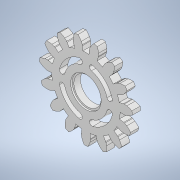
# Autodesk Inventor part: ｍ2歯数15ギア3td3.99
Saved by Autodesk Inventor 2020.2 (Build 242310000, 310)
## iProperties
Created: 2020-03-08
Part Number: ｍ2歯数15ギア3td3.99
Material: アルミニウム 2014-T4
Document SubType Name: Modeling
Designer: aoyam
Density: 2.8 g/cm^3
Appearance: サテン
Author: aoyam
Autodesk Inventor part; units mm, degrees
ref_plane "YZ Plane" through (0, 0, 0) normal (1, 0, 0) x (0, 1, 0)
ref_plane "XZ Plane" through (0, 0, 0) normal (0, 1, 0) x (-1, 0, 0)
ref_plane "XY Plane" through (0, 0, 0) normal (0, 0, 1) x (1, 0, 0)
sketch "スケッチ1" plane through (0, 0, 0) normal (0, 0, 1) x (1, 0, 0)
  arc A0 (3.0837, 16.0363) -> (3.0209, 15.76) centre (4.5944, 15.5478) ccw
  arc A1 (3.4621, 16.9034) -> (3.0837, 16.0363) centre (7.2791, 14.7216) ccw
  arc A2 (4.6507, 18.4808) -> (3.4621, 16.9034) centre (10.1692, 13.0859) ccw
  arc A3 (0.486, 15.76) -> (0.4232, 16.0363) centre (-1.0874, 15.5478) ccw
  arc A4 (0.4232, 16.0363) -> (0.0449, 16.9034) centre (-3.7722, 14.7216) ccw
  arc A5 (0.0449, 16.9034) -> (-1.1438, 18.4808) centre (-6.6623, 13.0859) ccw
  arc A6 (2.8775, 14.1671) -> (0.6295, 14.1671) centre (1.7535, 1.6862) ccw
  arc A7 (-1.1438, 18.4808) -> (-2.4308, 18.2073) centre (1.7535, 1.6862) ccw
  line L0 (2.8775, 14.1671) -> (3.0209, 15.76)
  line L1 (0.6295, 14.1671) -> (0.486, 15.76)
  line L2 (-4.3498, 12.6309) -> (-5.1288, 14.0278)
  arc A8 (-5.1288, 14.0278) -> (-5.2985, 14.2546) centre (-6.4799, 13.1939) ccw
  arc A9 (-5.2985, 14.2546) -> (-5.9968, 14.8928) centre (-8.5965, 11.3472) ccw
  arc A10 (-5.9968, 14.8928) -> (-7.7243, 15.8504) centre (-10.5714, 8.6774) ccw
  arc A11 (-7.7243, 15.8504) -> (-8.7887, 15.0771) centre (1.7535, 1.6862) ccw
  arc A12 (-2.868, 15.3367) -> (-2.813, 15.0588) centre (-1.2893, 15.5049) ccw
  arc A13 (-2.2961, 13.5452) -> (-4.3498, 12.6309) centre (1.7535, 1.6862) ccw
  line L3 (-2.2961, 13.5452) -> (-2.813, 15.0588)
  arc A14 (-2.875, 16.2827) -> (-2.868, 15.3367) centre (1.4994, 15.8421) ccw
  arc A15 (-2.4308, 18.2073) -> (-2.875, 16.2827) centre (4.805, 15.5234) ccw
  line L4 (-8.2737, 9.2022) -> (-9.5535, 10.1615)
  arc A16 (-9.5535, 10.1615) -> (-9.8008, 10.2997) centre (-10.4487, 8.8502) ccw
  arc A17 (-9.8008, 10.2997) -> (-10.6984, 10.5987) centre (-11.6311, 6.3022) ccw
  arc A18 (-10.6984, 10.5987) -> (-12.666, 10.7709) centre (-12.3494, 3.06) ccw
  arc A19 (-12.666, 10.7709) -> (-13.3239, 9.6314) centre (1.7535, 1.6862) ccw
  arc A20 (-8.0207, 12.2768) -> (-7.8573, 12.0453) centre (-6.6468, 13.0726) ccw
  arc A21 (-6.7695, 10.8728) -> (-8.2737, 9.2022) centre (1.7535, 1.6862) ccw
  line L5 (-6.7695, 10.8728) -> (-7.8573, 12.0453)
  arc A22 (-8.4118, 13.1382) -> (-8.0207, 12.2768) centre (-4.2364, 14.515) ccw
  arc A23 (-8.7887, 15.0771) -> (-8.4118, 13.1382) centre (-1.0869, 15.5682) ccw
  line L6 (-10.4639, 4.474) -> (-12.0232, 4.8298)
  arc A24 (-12.0232, 4.8298) -> (-12.3054, 4.8555) centre (-12.3076, 3.2678) ccw
  arc A25 (-12.3054, 4.8555) -> (-13.2469, 4.7636) centre (-12.3515, 0.4591) ccw
  arc A26 (-13.2469, 4.7636) -> (-15.1145, 4.1206) centre (-11.6889, -2.795) ccw
  arc A27 (-15.1145, 4.1206) -> (-15.252, 2.812) centre (1.7535, 1.6862) ccw
  arc A28 (-11.4832, 7.3857) -> (-11.2399, 7.2407) centre (-10.5518, 8.6715) ccw
  arc A29 (-9.7692, 6.612) -> (-10.4639, 4.474) centre (1.7535, 1.6862) ccw
  line L7 (-9.7692, 6.612) -> (-11.2399, 7.2407)
  arc A30 (-12.1909, 8.0135) -> (-11.4832, 7.3857) centre (-8.9365, 10.9696) ccw
  arc A31 (-13.3239, 9.6314) -> (-12.1909, 8.0135) centre (-6.4877, 13.2128) ccw
  line L8 (-10.5416, -0.7363) -> (-12.1108, -1.0455)
  arc A32 (-12.1108, -1.0455) -> (-12.379, -1.1368) centre (-11.7353, -2.5881) ccw
  arc A33 (-12.379, -1.1368) -> (-13.2018, -1.6037) centre (-10.633, -5.1718) ccw
  arc A34 (-13.2018, -1.6037) -> (-14.6463, -2.9507) centre (-8.7041, -7.8751) ccw
  arc A35 (-14.6463, -2.9507) -> (-14.2397, -4.2021) centre (1.7535, 1.6862) ccw
  arc A36 (-12.6571, 1.5091) -> (-12.3758, 1.4756) centre (-12.3292, 3.0626) ccw
  arc A37 (-10.7765, 1.4994) -> (-10.5416, -0.7363) centre (1.7535, 1.6862) ccw
  line L9 (-10.7765, 1.4994) -> (-12.3758, 1.4756)
  arc A38 (-13.5589, 1.7948) -> (-12.6571, 1.5091) centre (-11.7881, 5.819) ccw
  arc A39 (-15.252, 2.812) -> (-13.5589, 1.7948) centre (-10.4635, 8.8642) ccw
  line L10 (-8.4933, -5.5277) -> (-9.8011, -6.4484)
  arc A40 (-9.8011, -6.4484) -> (-10.009, -6.6409) centre (-8.8306, -7.705) ccw
  arc A41 (-10.009, -6.6409) -> (-10.5707, -7.4021) centre (-6.7727, -9.6169) ccw
  arc A42 (-10.5707, -7.4021) -> (-11.3425, -9.2202) centre (-3.9111, -11.302) ccw
  arc A43 (-11.3425, -9.2202) -> (-10.4621, -10.198) centre (1.7535, 1.6862) ccw
  arc A44 (-11.3392, -4.3369) -> (-11.0686, -4.2531) centre (-11.6715, -2.7843) ccw
  arc A45 (-9.6173, -3.5809) -> (-8.4933, -5.5277) centre (1.7535, 1.6862) ccw
  line L11 (-9.6173, -3.5809) -> (-11.0686, -4.2531)
  arc A46 (-12.2793, -4.4427) -> (-11.3392, -4.3369) centre (-12.2984, -0.0462) ccw
  arc A47 (-14.2397, -4.2021) -> (-12.2793, -4.4427) centre (-12.3269, 3.2746) ccw
  line L12 (-4.6733, -9.0717) -> (-5.4935, -10.4448)
  arc A48 (-5.4935, -10.4448) -> (-5.6051, -10.7052) centre (-4.0958, -11.198) ccw
  arc A49 (-5.6051, -10.7052) -> (-5.8087, -11.6291) centre (-1.4382, -12.1076) ccw
  arc A50 (-5.8087, -11.6291) -> (-5.7743, -13.6039) centre (1.8614, -12.4831) ccw
  arc A51 (-5.7743, -13.6039) -> (-4.5723, -14.1391) centre (1.7535, 1.6862) ccw
  arc A52 (-7.7575, -9.1414) -> (-7.5443, -8.9548) centre (-8.6925, -7.8583) ccw
  arc A53 (-6.4919, -7.7504) -> (-4.6733, -9.0717) centre (1.7535, 1.6862) ccw
  line L13 (-6.4919, -7.7504) -> (-7.5443, -8.9548)
  arc A54 (-8.5732, -9.6205) -> (-7.7575, -9.1414) centre (-10.3789, -5.6118) ccw
  arc A55 (-10.4621, -10.198) -> (-8.5732, -9.6205) centre (-11.7556, -2.5898) ccw
  line L14 (0.258, -10.7557) -> (0.0671, -12.3436)
  arc A56 (0.0671, -12.3436) -> (0.0711, -12.6269) centre (1.6503, -12.4632) ccw
  arc A57 (0.0711, -12.6269) -> (0.2609, -13.5537) centre (4.4482, -12.2133) ccw
  arc A58 (0.2609, -13.5537) -> (1.0956, -15.3438) centre (7.6152, -11.2142) ccw
  arc A59 (1.0956, -15.3438) -> (2.4114, -15.3438) centre (1.7535, 1.6862) ccw
  arc A60 (-2.5312, -12.0738) -> (-2.4124, -11.8166) centre (-3.9074, -11.2819) ccw
  arc A61 (-1.9409, -10.2883) -> (0.258, -10.7557) centre (1.7535, 1.6862) ccw
  line L15 (-1.9409, -10.2883) -> (-2.4124, -11.8166)
  arc A62 (-3.0816, -12.8432) -> (-2.5312, -12.0738) centre (-6.3616, -9.9156) ccw
  arc A63 (-4.5723, -14.1391) -> (-3.0816, -12.8432) centre (-8.8485, -7.7147) ccw
  line L16 (5.4478, -10.2883) -> (5.9194, -11.8166)
  arc A64 (5.9194, -11.8166) -> (6.0382, -12.0738) centre (7.4143, -11.2819) ccw
  arc A65 (6.0382, -12.0738) -> (6.5886, -12.8432) centre (9.8686, -9.9156) ccw
  arc A66 (6.5886, -12.8432) -> (8.0792, -14.1391) centre (12.3555, -7.7147) ccw
  arc A67 (8.0792, -14.1391) -> (9.2812, -13.6039) centre (1.7535, 1.6862) ccw
  arc A68 (3.4359, -12.6269) -> (3.4398, -12.3436) centre (1.8566, -12.4632) ccw
  arc A69 (3.249, -10.7557) -> (5.4478, -10.2883) centre (1.7535, 1.6862) ccw
  line L17 (3.249, -10.7557) -> (3.4398, -12.3436)
  arc A70 (3.2461, -13.5537) -> (3.4359, -12.6269) centre (-0.9412, -12.2133) ccw
  arc A71 (2.4114, -15.3438) -> (3.2461, -13.5537) centre (-4.1082, -11.2142) ccw
  line L18 (9.9989, -7.7504) -> (11.0513, -8.9548)
  arc A72 (11.0513, -8.9548) -> (11.2644, -9.1414) centre (12.1995, -7.8583) ccw
  arc A73 (11.2644, -9.1414) -> (12.0802, -9.6205) centre (13.8859, -5.6118) ccw
  arc A74 (12.0802, -9.6205) -> (13.969, -10.198) centre (15.2626, -2.5898) ccw
  arc A75 (13.969, -10.198) -> (14.8494, -9.2202) centre (1.7535, 1.6862) ccw
  arc A76 (9.1121, -10.7052) -> (9.0005, -10.4448) centre (7.6028, -11.198) ccw
  arc A77 (8.1802, -9.0717) -> (9.9989, -7.7504) centre (1.7535, 1.6862) ccw
  line L19 (8.1802, -9.0717) -> (9.0005, -10.4448)
  arc A78 (9.3156, -11.6291) -> (9.1121, -10.7052) centre (4.9452, -12.1076) ccw
  arc A79 (9.2812, -13.6039) -> (9.3156, -11.6291) centre (1.6456, -12.4831) ccw
  line L20 (13.1242, -3.5809) -> (14.5755, -4.2531)
  arc A80 (14.5755, -4.2531) -> (14.8462, -4.3369) centre (15.1785, -2.7843) ccw
  arc A81 (14.8462, -4.3369) -> (15.7862, -4.4427) centre (15.8053, -0.0462) ccw
  arc A82 (15.7862, -4.4427) -> (17.7467, -4.2021) centre (15.8338, 3.2746) ccw
  arc A83 (17.7467, -4.2021) -> (18.1533, -2.9507) centre (1.7535, 1.6862) ccw
  arc A84 (13.5159, -6.6409) -> (13.3081, -6.4484) centre (12.3375, -7.705) ccw
  arc A85 (12.0002, -5.5277) -> (13.1242, -3.5809) centre (1.7535, 1.6862) ccw
  line L21 (12.0002, -5.5277) -> (13.3081, -6.4484)
  arc A86 (14.0777, -7.4021) -> (13.5159, -6.6409) centre (10.2797, -9.6169) ccw
  arc A87 (14.8494, -9.2202) -> (14.0777, -7.4021) centre (7.4181, -11.302) ccw
  line L22 (14.2835, 1.4994) -> (15.8827, 1.4756)
  arc A88 (15.8827, 1.4756) -> (16.164, 1.5091) centre (15.8361, 3.0626) ccw
  arc A89 (16.164, 1.5091) -> (17.0659, 1.7948) centre (15.2951, 5.819) ccw
  arc A90 (17.0659, 1.7948) -> (18.759, 2.812) centre (13.9705, 8.8642) ccw
  arc A91 (18.759, 2.812) -> (18.6214, 4.1206) centre (1.7535, 1.6862) ccw
  arc A92 (15.8859, -1.1368) -> (15.6177, -1.0455) centre (15.2422, -2.5881) ccw
  arc A93 (14.0485, -0.7363) -> (14.2835, 1.4994) centre (1.7535, 1.6862) ccw
  line L23 (14.0485, -0.7363) -> (15.6177, -1.0455)
  arc A94 (16.7087, -1.6037) -> (15.8859, -1.1368) centre (14.1399, -5.1718) ccw
  arc A95 (18.1533, -2.9507) -> (16.7087, -1.6037) centre (12.2111, -7.8751) ccw
  line L24 (13.2762, 6.612) -> (14.7468, 7.2407)
  arc A96 (14.7468, 7.2407) -> (14.9902, 7.3857) centre (14.0588, 8.6715) ccw
  arc A97 (14.9902, 7.3857) -> (15.6979, 8.0135) centre (12.4434, 10.9696) ccw
  arc A98 (15.6979, 8.0135) -> (16.8308, 9.6314) centre (9.9947, 13.2128) ccw
  arc A99 (16.8308, 9.6314) -> (16.173, 10.7709) centre (1.7535, 1.6862) ccw
  arc A100 (15.8123, 4.8555) -> (15.5302, 4.8298) centre (15.8146, 3.2678) ccw
  arc A101 (13.9708, 4.474) -> (13.2762, 6.612) centre (1.7535, 1.6862) ccw
  line L25 (13.9708, 4.474) -> (15.5302, 4.8298)
  arc A102 (16.7539, 4.7636) -> (15.8123, 4.8555) centre (15.8584, 0.4591) ccw
  arc A103 (18.6214, 4.1206) -> (16.7539, 4.7636) centre (15.1959, -2.795) ccw
  line L26 (10.2765, 10.8728) -> (11.3643, 12.0453)
  arc A104 (11.3643, 12.0453) -> (11.5276, 12.2768) centre (10.1537, 13.0726) ccw
  arc A105 (11.5276, 12.2768) -> (11.9188, 13.1382) centre (7.7433, 14.515) ccw
  arc A106 (11.9188, 13.1382) -> (12.2957, 15.0771) centre (4.5939, 15.5682) ccw
  arc A107 (12.2957, 15.0771) -> (11.2312, 15.8504) centre (1.7535, 1.6862) ccw
  arc A108 (13.3078, 10.2997) -> (13.0605, 10.1615) centre (13.9556, 8.8502) ccw
  arc A109 (11.7807, 9.2022) -> (10.2765, 10.8728) centre (1.7535, 1.6862) ccw
  line L27 (11.7807, 9.2022) -> (13.0605, 10.1615)
  arc A110 (14.2053, 10.5987) -> (13.3078, 10.2997) centre (15.1381, 6.3022) ccw
  arc A111 (16.173, 10.7709) -> (14.2053, 10.5987) centre (15.8564, 3.06) ccw
  line L28 (5.8031, 13.5452) -> (6.3199, 15.0588)
  arc A112 (6.3199, 15.0588) -> (6.375, 15.3367) centre (4.7962, 15.5049) ccw
  arc A113 (6.375, 15.3367) -> (6.382, 16.2827) centre (2.0075, 15.8421) ccw
  arc A114 (6.382, 16.2827) -> (5.9377, 18.2073) centre (-1.298, 15.5234) ccw
  arc A115 (5.9377, 18.2073) -> (4.6507, 18.4808) centre (1.7535, 1.6862) ccw
  arc A116 (8.8054, 14.2546) -> (8.6357, 14.0278) centre (9.9868, 13.1939) ccw
  arc A117 (7.8567, 12.6309) -> (5.8031, 13.5452) centre (1.7535, 1.6862) ccw
  line L29 (7.8567, 12.6309) -> (8.6357, 14.0278)
  arc A118 (9.5037, 14.8928) -> (8.8054, 14.2546) centre (12.1034, 11.3472) ccw
  arc A119 (11.2312, 15.8504) -> (9.5037, 14.8928) centre (14.0783, 8.6774) ccw
  circle A120 centre (1.7535, 1.6862) radius 5
  point P0 (0, 0)
  point P1 (10.2765, 10.8728)
  point P2 (11.3643, 12.0453)
  point P3 (11.5276, 12.2768)
  point P4 (11.9188, 13.1382)
  point P5 (12.2957, 15.0771)
  point P6 (11.2312, 15.8504)
  point P7 (9.5037, 14.8928)
  point P8 (8.8054, 14.2546)
  point P9 (5.8031, 13.5452)
  point P10 (6.3199, 15.0588)
  point P11 (6.375, 15.3367)
  point P12 (6.382, 16.2827)
  point P13 (5.9377, 18.2073)
  point P14 (4.6507, 18.4808)
  point P15 (3.4621, 16.9034)
  point P16 (3.0837, 16.0363)
  point P17 (2.8775, 14.1671)
  point P18 (0.6295, 14.1671)
  point P19 (0.4232, 16.0363)
  point P20 (0.0449, 16.9034)
  point P21 (-1.1438, 18.4808)
  point P22 (-2.4308, 18.2073)
  point P23 (-2.875, 16.2827)
  point P24 (-2.868, 15.3367)
  point P25 (-5.2985, 14.2546)
  point P26 (-5.9968, 14.8928)
  point P27 (-7.7243, 15.8504)
  point P28 (-8.7887, 15.0771)
  point P29 (-8.4118, 13.1382)
  point P30 (-8.0207, 12.2768)
  point P31 (-7.8573, 12.0453)
  point P32 (-6.7695, 10.8728)
  point P33 (-9.8008, 10.2997)
  point P34 (-10.6984, 10.5987)
  point P35 (-12.666, 10.7709)
  point P36 (-13.3239, 9.6314)
  point P37 (-12.1909, 8.0135)
  point P38 (-11.4832, 7.3857)
  point P39 (-12.0232, 4.8298)
  point P40 (-12.3054, 4.8555)
  point P41 (-13.2469, 4.7636)
  point P42 (-15.1145, 4.1206)
  point P43 (-15.252, 2.812)
  point P44 (-13.5589, 1.7948)
  point P45 (-12.6571, 1.5091)
  point P46 (-12.3758, 1.4756)
  point P47 (-10.7765, 1.4994)
  point P48 (-12.379, -1.1368)
  point P49 (-13.2018, -1.6037)
  point P50 (-14.6463, -2.9507)
  point P51 (-14.2397, -4.2021)
  point P52 (-12.2793, -4.4427)
  point P53 (-11.3392, -4.3369)
  point P54 (-9.6173, -3.5809)
  point P55 (-8.4933, -5.5277)
  point P56 (-9.8011, -6.4484)
  point P57 (-10.009, -6.6409)
  point P58 (-10.5707, -7.4021)
  point P59 (-11.3425, -9.2202)
  point P60 (-10.4621, -10.198)
  point P61 (-8.5732, -9.6205)
  point P62 (-7.7575, -9.1414)
  point P63 (-7.5443, -8.9548)
  point P64 (-5.6051, -10.7052)
  point P65 (-5.8087, -11.6291)
  point P66 (-5.7743, -13.6039)
  point P67 (-4.5723, -14.1391)
  point P68 (-3.0816, -12.8432)
  point P69 (-2.5312, -12.0738)
  point P70 (0.258, -10.7557)
  point P71 (0.0711, -12.6269)
  point P72 (0.2609, -13.5537)
  point P73 (1.0956, -15.3438)
  point P74 (2.4114, -15.3438)
  point P75 (3.2461, -13.5537)
  point P76 (3.4359, -12.6269)
  point P77 (5.4478, -10.2883)
  point P78 (5.9194, -11.8166)
  point P79 (6.0382, -12.0738)
  point P80 (6.5886, -12.8432)
  point P81 (8.0792, -14.1391)
  point P82 (9.2812, -13.6039)
  point P83 (9.3156, -11.6291)
  point P84 (9.1121, -10.7052)
  point P85 (9.9989, -7.7504)
  point P86 (11.0513, -8.9548)
  point P87 (12.0802, -9.6205)
  point P88 (13.969, -10.198)
  point P89 (14.8494, -9.2202)
  point P90 (14.0777, -7.4021)
  point P91 (13.5159, -6.6409)
  point P92 (13.1242, -3.5809)
  point P93 (14.5755, -4.2531)
  point P94 (14.8462, -4.3369)
  point P95 (15.7862, -4.4427)
  point P96 (17.7467, -4.2021)
  point P97 (18.1533, -2.9507)
  point P98 (16.7087, -1.6037)
  point P99 (15.8859, -1.1368)
  point P100 (14.2835, 1.4994)
  point P101 (15.8827, 1.4756)
  point P102 (16.164, 1.5091)
  point P103 (17.0659, 1.7948)
  point P104 (18.759, 2.812)
  point P105 (18.6214, 4.1206)
  point P106 (16.7539, 4.7636)
  point P107 (15.8123, 4.8555)
  point P108 (13.2762, 6.612)
  point P109 (14.7468, 7.2407)
  point P110 (15.6979, 8.0135)
  point P111 (16.8308, 9.6314)
  point P112 (16.173, 10.7709)
  point P113 (14.2053, 10.5987)
  point P114 (13.3078, 10.2997)
  dimension "d2" = 360
  dimension "d4" = 10
  dimension "d21" = 12.5314
  constraints: 240 point on circle, 121 centre point, 60 end point, 3 coincident, 569 other
  measures "d4" diameter of A120
  measures "d21" radius of A21
extrude "押し出し1" add sketch "スケッチ1" along normal blind 3
sketch "スケッチ2" plane through (0, 0, 3) normal (0, 0, 1) x (1, 0, 0)
  circle A0 centre (1.7535, 1.6862) radius 5 projected
  circle A1 centre (1.7535, 1.6862) radius 12.5
  circle A2 centre (1.7535, 1.6862) radius 10
  circle A3 centre (1.7535, 1.6862) radius 8
  line L0 (-8.2465, 1.6862) -> (-6.2465, 1.6862) construction
  line L1 (-8.2465, 0.959) -> (-6.2465, 0.959)
  line L2 (-6.2465, 2.959) -> (-8.2465, 2.959)
  line L3 (-8.2465, 1.6862) -> (-7.2465, 1.6862) construction
  line L4 (-7.2465, 1.6862) -> (-2.2415, 1.6862) construction
  line L5 (-6.2465, 1.6862) -> (-2.2415, 1.6862)
  line L6 (-2.2415, 1.6862) -> (1.7535, 1.6862) construction
  arc A4 (-7.9206, 4.2185) -> (-6.9483, 2.959) centre (-6.9483, 3.964) ccw
  arc A5 (-6.9587, 2.959) -> (-5.9863, 3.7098) centre (-6.9587, 3.964) ccw
  arc A6 (-6.9483, 0.4133) -> (-7.9206, -0.8462) centre (-6.9483, -0.5917) ccw
  arc A7 (-5.9863, -0.3375) -> (-6.9587, 0.4133) centre (-6.9587, -0.5917) ccw
  arc A8 (-6.2465, 0.959) -> (-6.2135, 0.9598) centre (-6.2465, 1.6862) ccw
  arc A9 (-6.1453, 2.955) -> (-6.2465, 2.959) centre (-6.2465, 1.6862) ccw
  arc A10 (-0.7789, -7.9879) -> (0.4806, -7.0156) centre (-0.5244, -7.0156) ccw
  arc A11 (3.0263, -7.0156) -> (4.2858, -7.9879) centre (4.0313, -7.0156) ccw
  arc A12 (3.7771, -6.0536) -> (3.0263, -7.026) centre (4.0313, -7.026) ccw
  arc A13 (0.4806, -7.026) -> (-0.2702, -6.0536) centre (-0.5244, -7.026) ccw
  arc A14 (11.4275, -0.8462) -> (10.4553, 0.4133) centre (10.4553, -0.5917) ccw
  arc A15 (10.4553, 2.959) -> (11.4275, 4.2185) centre (10.4553, 3.964) ccw
  arc A16 (9.4933, 3.7098) -> (10.4656, 2.959) centre (10.4656, 3.964) ccw
  arc A17 (10.4656, 0.4133) -> (9.4933, -0.3375) centre (10.4656, -0.5917) ccw
  arc A18 (4.2858, 11.3602) -> (3.0263, 10.388) centre (4.0313, 10.388) ccw
  arc A19 (0.4806, 10.388) -> (-0.7789, 11.3602) centre (-0.5244, 10.388) ccw
  arc A20 (-0.2702, 9.426) -> (0.4806, 10.3983) centre (-0.5244, 10.3983) ccw
  arc A21 (3.0263, 10.3983) -> (3.7771, 9.426) centre (4.0313, 10.3983) ccw
  line L7 (0.4806, 10.3983) -> (0.4806, 10.388)
  line L8 (3.0263, 10.388) -> (3.0263, 10.3983)
  line L9 (10.4656, 2.959) -> (13.5792, 2.959)
  line L10 (10.4656, 0.4133) -> (10.4553, 0.4133)
  line L11 (0.4806, -7.026) -> (0.4806, -7.0156)
  line L12 (3.0263, -7.026) -> (3.0263, -7.0156)
  point P0 (0, 0)
  point P1 (3.7771, 9.426)
  point P2 (9.4933, 3.7098)
  point P3 (10.5222, 2.6862)
  point P4 (11.4275, 4.2185)
  point P5 (4.2858, 11.3602)
  point P6 (4.2858, -7.9879)
  point P7 (11.4275, -0.8462)
  point P8 (9.4933, -0.3375)
  point P9 (3.7771, -6.0536)
  point P10 (-0.2702, -6.0536)
  point P11 (-5.9863, -0.3375)
  point P12 (-3.9016, 0.6862)
  point P13 (-7.0152, 0.6862)
  point P14 (-7.9206, -0.8462)
  point P15 (-0.7789, -7.9879)
  point P16 (-0.7789, 11.3602)
  point P17 (-0.2702, 9.426)
  point P18 (3.0264, 10.3931)
  point P19 (10.4604, 2.9591)
  point P20 (10.4604, 0.4133)
  point P21 (3.0264, -7.0208)
  point P22 (0.4806, -7.0208)
  point P23 (-6.9535, 0.4133)
  point P24 (0.4806, 10.3931)
  point P25 (-6.9535, 2.9591)
  dimension "d7" = 25
  dimension "d8" = 2.5
  dimension "d9" = 3
  dimension "d11" = 2.01
  dimension "d12" = 2.01
  dimension "d15" = 360
  dimension "d19" = 2
  constraints: 42 point on circle, 28 end point, 21 centre point, 8 tangent, 6 symmetric about line, 5 horizontal, 2 parallel, 2 point on line, 2 vertical, 1 coincident, 1 collinear, 1 midpoint, 67 other
  measures "d7" diameter of A1
  measures "d8" radial gap between concentric circles of A1 A2
  measures "d9" radial gap between concentric circles of A0 A3
  measures "d11" diameter of A4
  measures "d12" diameter of A5
  measures "d19" distance between parallel lines of L1 L2
extrude "押し出し2" cut sketch "スケッチ2" against normal blind 3 contours A5 L2 A4 A2 A19 A20 A3 | A3 A13 A10 A2 A6 A7 | A21 A18 A2 A15 A16 A3 | A3 A17 A14 A2 A11 A12
sketch "スケッチ3" plane through (0, 0, 3) normal (0, 0, 1) x (1, 0, 0)
  circle A0 centre (1.7535, 1.6862) radius 5 projected
  circle A1 centre (1.7535, 1.6862) radius 5.6
  point P0 (0, 0)
  dimension "d22" = 0.6
  constraints: 1 centre point
  measures "d22" radial gap between concentric circles of A0 A1
extrude "押し出し3" cut sketch "スケッチ3" against normal blind 0.6
